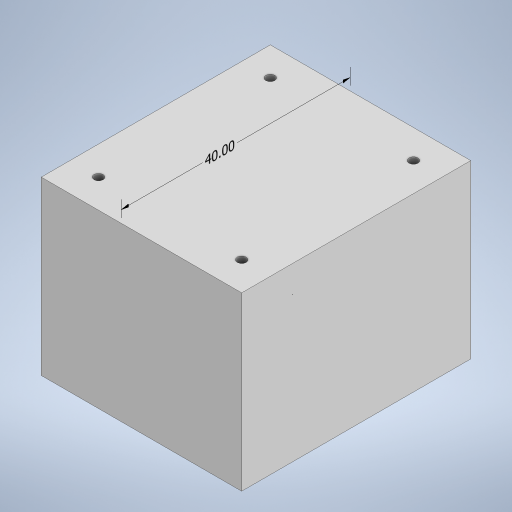
# Autodesk Inventor part: board
Saved by Autodesk Inventor 2024.1 (Build 281209000, 209)
## iProperties
Created: 2024-02-13
Part Number: board
Material: 一般
Document SubType Name: Modeling
Designer: hibik
Density: 1 g/cm^3
Appearance: 既定
Author: hibik
Autodesk Inventor part; units mm, degrees
ref_plane "YZ Plane" through (0, 0, 0) normal (1, 0, 0) x (0, 1, 0)
ref_plane "XZ Plane" through (0, 0, 0) normal (0, 1, 0) x (-1, 0, 0)
ref_plane "XY Plane" through (0, 0, 0) normal (0, 0, 1) x (1, 0, 0)
sketch "スケッチ1" plane through (0, 0, 0) normal (0, 1, 0) x (-1, 0, 0)
  line L0 (35, 0) -> (0, 0)
  line L1 (0, 0) -> (0, -40)
  line L2 (0, -40) -> (35, -40)
  line L3 (35, -40) -> (35, 0)
  line L4 (30, -5) -> (5, -5)
  line L5 (5, -5) -> (5, -35)
  line L6 (5, -35) -> (30, -35)
  line L7 (30, -35) -> (30, -5)
  circle A0 centre (30, -5) radius 0.8
  circle A1 centre (30, -35) radius 0.8
  circle A2 centre (5, -35) radius 0.8
  circle A3 centre (5, -5) radius 0.8
  dimension "d0" = 25
  dimension "d1" = 30
  dimension "d2" = 5
  dimension "d3" = 5
  dimension "d4" = 5
  dimension "d5" = 5
  dimension "d6" = 1.6
  dimension "d7" = 1.6
  dimension "d8" = 1.6
  dimension "d9" = 1.6
  constraints: 16 end point, 4 centre point, 4 coincident, 4 parallel, 2 horizontal, 2 perpendicular
  measures "d0" distance of L4.start L4.end
  measures "d1" distance of L4.end L5.end
  measures "d2" distance between parallel lines of L3 L7
  measures "d3" distance between parallel lines of L1 L5
  measures "d4" distance between parallel lines of L0 L4
  measures "d5" distance between parallel lines of L2 L6
  measures "d6" diameter of A0
  measures "d7" diameter of A1
  measures "d8" diameter of A2
  measures "d9" diameter of A3
extrude "押し出し1" add sketch "スケッチ1" along normal blind 30 contours L3 L2 L1 L0 | L4 A0 L7 A1 L6 A2 L5 A3
equation "\"d3\" = d2"
equation "\"d4\" = d2"
equation "\"d5\" = d2"
